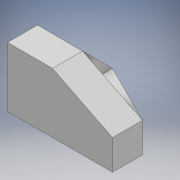
# Autodesk Inventor part: 13
Saved by Autodesk Inventor 2017 (Build 210142000, 142)
## iProperties
Part Number: 13
Material: 一般
Document SubType Name: Modeling
Designer: Brian
Density: 1 g/cm^3
Appearance: 預設
Author: Brian
Autodesk Inventor part; units mm, degrees
ref_plane "YZ Plane" through (0, 0, 0) normal (1, 0, 0) x (0, 1, 0)
ref_plane "XZ Plane" through (0, 0, 0) normal (0, 1, 0) x (-1, 0, 0)
ref_plane "XY Plane" through (0, 0, 0) normal (0, 0, 1) x (1, 0, 0)
sketch "草圖1" plane through (0, 0, 0) normal (0, 1, 0) x (-1, 0, 0)
  line L0 (0, 0) -> (-30, 0)
  line L1 (-30, 0) -> (-30, -20)
  line L2 (-30, -20) -> (0, -20)
  line L3 (0, -20) -> (0, 0)
  line L4 (0, -20) -> (-70, -20)
  line L5 (-70, -20) -> (-70, -40)
  line L6 (-70, -40) -> (0, -40)
  line L7 (0, -40) -> (0, -20)
  line L8 (-70, -20) -> (-30, 0)
  dimension "d0" = 70
  dimension "d1" = 20
  dimension "d2" = 20
  dimension "d3" = 30
  constraints: 18 end point, 4 parallel, 2 horizontal, 2 perpendicular
  measures "d0" distance of L5.end L6.end
  measures "d1" distance of L6.end L2.end
  measures "d2" distance of L2.end L0.start
  measures "d3" distance of L0.start L0.end
extrude "擠出1" add sketch "草圖1" along normal blind 20
sketch "草圖2" plane through (0, 0, -40) normal (-1, 0, 0) x (0, 0, 1)
  line L0 (0, 0) -> (0, 20) projected
  line L1 (0, 20) -> (20, 20)
  line L2 (20, 20) -> (20, 40)
  line L3 (20, 40) -> (0, 40)
  line L4 (0, 40) -> (0, 20)
  line L5 (20, 40) -> (40, 20)
  line L6 (40, 20) -> (20, 20)
  line L7 (40, 20) -> (20, 20) projected
  point P0 (40, 0)
  dimension "d6" = 20
  dimension "d7" = 20
  constraints: 12 end point, 3 equal length, 1 horizontal, 1 perpendicular
  measures "d6" distance of L2.end L3.end
  measures "d7" distance of L3.end L0.end
extrude "擠出2" add sketch "草圖2" against normal blind 30
sketch "草圖3" plane through (70, 0, -40) normal (0, 0, -1) x (-1, 0, 0)
  line L0 (40, 20) -> (40, 40) projected
  line L1 (0, 20) -> (40, 20) projected
  line L2 (0, 20) -> (40, 40)
  point P0 (70, 0)
  constraints: 2 end point
extrude "擠出3" add sketch "草圖3" against normal blind 20
